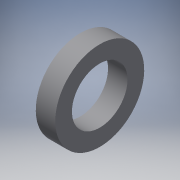
# Autodesk Inventor part: 6804
Saved by Autodesk Inventor 2019.4 (Build 234330000, 330)
## iProperties
Created: 2019-12-12
Part Number: 6804
Material: Generic
Document SubType Name: Modeling
Designer: Mark
Density: 1 g/cm^3
Appearance: Default
Author: Mark
Autodesk Inventor part; units mm, degrees
ref_plane "YZ Plane" through (0, 0, 0) normal (1, 0, 0) x (0, 1, 0)
ref_plane "XZ Plane" through (0, 0, 0) normal (0, 1, 0) x (-1, 0, 0)
ref_plane "XY Plane" through (0, 0, 0) normal (0, 0, 1) x (1, 0, 0)
sketch "Sketch1" plane through (0, 0, 0) normal (1, 0, 0) x (0, 1, 0)
  circle A0 centre (0, 0) radius 10
  circle A1 centre (0, 0) radius 16
  line L0 (0, 0) -> (-20, 0) construction
  line L1 (0, 0) -> (20, 0) construction
  circle A2 centre (-23.5, 0) radius 3.5 construction
  circle A3 centre (-23.5, 0) radius 2.75
  circle A4 centre (-23.5, 0) radius 5
  circle A5 centre (0, 0) radius 20
  line L2 (-26.6915, -3.8489) -> (-12.766, -15.3958)
  line L3 (-26.6915, 3.8489) -> (-12.766, 15.3958)
  circle A6 centre (0, -20) radius 2.75
  circle A7 centre (0, -20) radius 4
  line L4 (0, 0) -> (0, -30) construction
  line L5 (2.4, -23.2) -> (12, -16)
  line L6 (-2.4, -23.2) -> (-12, -16)
  circle A8 centre (0, 20) radius 2.75
  circle A9 centre (0, 20) radius 4
  line L7 (2.4, 23.2) -> (12, 16)
  line L8 (-2.4, 23.2) -> (-12, 16)
  dimension "d6" = 7
  dimension "d8" = 10
  dimension "d0" = 20
  dimension "d1" = 32
  dimension "d4" = 20
  dimension "d5" = 180
  dimension "d7" = 5.5
  dimension "d9" = 40
  dimension "d10" = 5.5
  dimension "d11" = 30
  constraints: 18 end point, 8 centre point, 8 point on circle, 8 symmetric about line, 7 coincident, 6 tangent, 2 horizontal, 2 point on line, 1 collinear, 1 horizontal alignment, 1 vertical, 8 other
  measures "d0" diameter of A0
  measures "d1" diameter of A1
  measures "d4" distance of L0.start L0.end
  measures "d5" angle of L0 L1
  measures "d7" diameter of A3
  measures "d9" diameter of A5
  measures "d10" diameter of A6
  measures "d11" distance of L4.start L4.end
extrude "Extrusion1" add sketch "Sketch1" along normal blind 7 contours A1
body "Solid1"
